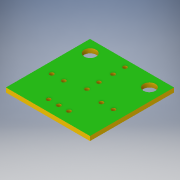
# Autodesk Inventor part: PCB_Sen_Color
Saved by Autodesk Inventor 2016 (Build 200138000, 138)
## iProperties
Created: 2016-04-16
Part Number: PCB_Sen_Color
Material: ABS Plastic
Document SubType Name: Modeling
Designer: Nanjar
Density: 1.06 g/cm^3
Appearance: Smooth - White
Author: Nanjar
Autodesk Inventor part; units mm, degrees
ref_plane "YZ Plane" through (0, 0, 0) normal (1, 0, 0) x (0, 1, 0)
ref_plane "XZ Plane" through (0, 0, 0) normal (0, 1, 0) x (-1, 0, 0)
ref_plane "XY Plane" through (0, 0, 0) normal (0, 0, 1) x (1, 0, 0)
sketch "Sketch1" plane through (0, 0, 0) normal (0, 1, 0) x (-1, 0, 0)
  line L0 (-10.5, -10.5) -> (10.5, -10.5)
  line L1 (10.5, -10.5) -> (10.5, 10.5)
  line L2 (10.5, 10.5) -> (-10.5, 10.5)
  line L3 (-10.5, 10.5) -> (-10.5, -10.5)
  line L4 (-10.5, -10.5) -> (10.5, 10.5) construction
  line L5 (10.5, -10.5) -> (-10.5, 10.5) construction
  point P0 (0, 0)
  dimension "d0" = 21
  dimension "d1" = 21
  constraints: 12 end point, 2 midpoint, 2 parallel, 1 horizontal, 1 perpendicular
  measures "d0" distance of L0.end L1.end
  measures "d1" distance of L1.end L2.end
extrude "Extrusion1" add sketch "Sketch1" along normal blind 1.1
sketch "Sketch2" plane through (0, 1.1, 0) normal (0, 1, 0) x (1, 0, 0)
  circle A0 centre (-7.4, 7.45) radius 1.5
  circle A1 centre (7.4, 7.45) radius 1.5
  circle A2 centre (0, 8.75) radius 0.5
  circle A3 centre (0, 5.75) radius 0.5
  circle A4 centre (-2.58, -7.75) radius 0.5
  circle A5 centre (-0.04, -7.75) radius 0.5
  circle A6 centre (2.5, -7.75) radius 0.5
  circle A7 centre (-7.7, -1.85) radius 0.5
  circle A8 centre (-4.7, -1.85) radius 0.5
  circle A9 centre (0, 2.25) radius 0.5
  circle A10 centre (0, -0.75) radius 0.5
  circle A11 centre (4.7, -1.85) radius 0.5
  circle A12 centre (7.7, -1.85) radius 0.5
  point P0 (0, 0)
  dimension "d4" = 3
  dimension "d5" = 3
  dimension "d10" = 1
  dimension "d12" = 1
  dimension "d14" = 1
  dimension "d15" = 1
  dimension "d16" = 1
  dimension "d23" = 2.54
  dimension "d24" = 2.54
  dimension "d25" = 1
  dimension "d27" = 1
  dimension "d28" = 3
  dimension "d31" = 1
  dimension "d32" = 1
  dimension "d36" = 3
  dimension "d37" = 1
  dimension "d38" = 1
  dimension "d40" = 3
  constraints: 13 centre point
  measures "d4" diameter of A0
  measures "d5" diameter of A1
  measures "d10" diameter of A2
  measures "d12" diameter of A3
  measures "d14" diameter of A4
  measures "d15" diameter of A5
  measures "d16" diameter of A6
  measures "d23" distance of A5.centre A4.centre
  measures "d24" distance of A6.centre A5.centre
  measures "d25" diameter of A7
  measures "d27" diameter of A8
  measures "d28" distance of A8.centre A7.centre
  measures "d31" diameter of A9
  measures "d32" diameter of A10
  measures "d36" distance of A10.centre A9.centre
  measures "d37" diameter of A11
  measures "d38" diameter of A12
  measures "d40" distance of A11.centre A12.centre
extrude "Extrusion2" cut sketch "Sketch2" against normal up to next
body "Solid1"
